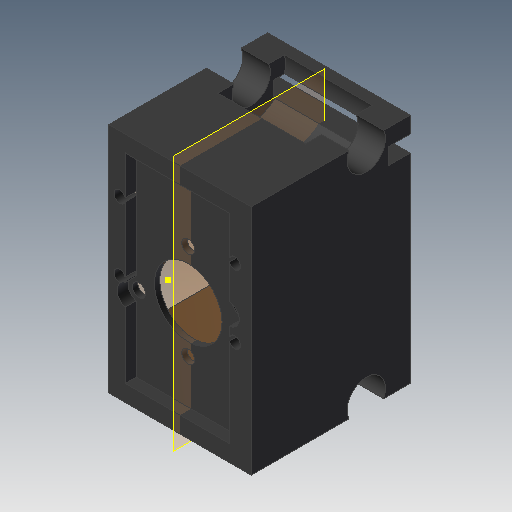
# Autodesk Inventor part: 01_Adapter_Raspicam_CCTV_lens
Saved by Autodesk Inventor 2019.4 (Build 234330000, 330)
## iProperties
Created: 2020-10-20
Part Number: 01_Adapter_Raspicam_CCTV_lens
Material: Generic
Document SubType Name: Modeling
Designer: diederichbenedict
Density: 1 g/cm^3
Appearance: Default
Author: diederichbenedict
Autodesk Inventor part; units mm, degrees
ref_plane "YZ Plane" through (0, 0, 0) normal (1, 0, 0) x (0, 1, 0)
ref_plane "XZ Plane" through (0, 0, 0) normal (0, 1, 0) x (-1, 0, 0)
ref_plane "Work Plane1" through (3.9765, -1.598, 6) normal (0, 0, 1) x (1, 0, 0)
sketch "Sketch1" plane through (3.9765, -1.598, 6) normal (0, 0, 1) x (1, 0, 0)
  arc A0 (8.7735, 0.8133) -> (8.7735, -0.0173) centre (8.2735, 0.398) ccw construction
  line L0 (8.7735, 0.8133) -> (8.7735, 2.1739) construction
  arc A1 (8.7735, 2.1739) -> (8.7735, 5.6221) centre (9.0735, 3.898) ccw construction
  line L1 (8.7735, 5.6221) -> (8.7735, 7.898) construction
  line L2 (8.7735, 7.898) -> (1.2743, 7.898) construction
  arc A2 (1.2743, 7.898) -> (-1.7274, 7.898) centre (-0.2265, 8.798) ccw construction
  line L3 (-1.7274, 7.898) -> (-8.2265, 7.898) construction
  line L4 (-8.2265, 7.898) -> (-8.2265, -1.1658) construction
  arc A3 (-8.2265, -1.1658) -> (-8.2265, -4.0381) centre (-9.2265, -2.602) ccw construction
  line L5 (-8.2265, -4.0381) -> (-8.2265, -8.102) construction
  line L6 (-8.2265, -8.102) -> (-1.9036, -8.102) construction
  arc A4 (-1.9036, -8.102) -> (1.4505, -8.102) centre (-0.2265, -8.602) ccw construction
  line L7 (1.4505, -8.102) -> (8.7735, -8.102) construction
  line L8 (8.7735, -8.102) -> (8.7735, -0.0173) construction
  line L9 (-6.2265, -6.102) -> (-6.2265, 5.898) construction
  line L10 (-6.2265, 5.898) -> (6.7735, 5.898) construction
  line L11 (6.7735, 5.898) -> (6.7735, -6.102) construction
  line L12 (6.7735, -6.102) -> (-6.2265, -6.102) construction
  circle A5 centre (-9.2265, -2.602) radius 0.9 construction
  circle A6 centre (9.0735, 3.898) radius 0.9 construction
  circle A7 centre (-0.2265, 8.798) radius 0.9 construction
  circle A8 centre (-0.2265, -8.602) radius 0.9 construction
  line L13 (10.1735, -9.602) -> (10.1735, -4.102) construction
  line L14 (12.2735, -9.602) -> (10.1735, -9.602) construction
  line L15 (12.2735, 14.398) -> (12.2735, -9.602) construction
  line L16 (-12.7265, 14.398) -> (12.2735, 14.398) construction
  line L17 (-12.7265, -9.602) -> (-12.7265, 14.398) construction
  line L18 (-10.6265, -9.602) -> (-12.7265, -9.602) construction
  line L19 (-10.6265, -4.102) -> (-10.6265, -9.602) construction
  line L20 (10.1735, -4.102) -> (-10.6265, -4.102) construction
  circle A9 centre (10.2735, 12.398) radius 1.05 construction
  circle A10 centre (10.2735, -0.102) radius 1.05 construction
  circle A11 centre (-10.7265, -0.102) radius 1.05 construction
  circle A12 centre (-10.7265, 12.398) radius 1.05 construction
  line L21 (8.7735, 0.798) -> (8.7735, 12.398) construction
  line L22 (-8.9265, 0.798) -> (8.7735, 0.798) construction
  line L23 (-8.9265, 12.398) -> (-8.9265, 0.798) construction
  line L24 (8.7735, 12.398) -> (-8.9265, 12.398) construction
  line L25 (12.2735, 14.398) -> (-12.7265, 14.398)
  line L26 (-12.7265, 14.398) -> (-12.7265, -9.602)
  line L27 (12.2735, -9.602) -> (12.2735, 14.398)
  circle A13 centre (-0.2265, 8.798) radius 1.2
  circle A14 centre (-9.2265, -2.602) radius 1.2
  circle A15 centre (-0.2265, -8.602) radius 1.2
  circle A16 centre (9.0735, 3.898) radius 1.2
  circle A17 centre (-0.2265, -0.102) radius 2.8 projected
  circle A18 centre (-0.2265, -0.102) radius 6.1789
  line L28 (-12.7265, -9.602) -> (-12.7265, -19.602)
  line L29 (-12.7265, -19.602) -> (12.2735, -19.602)
  line L30 (12.2735, -19.602) -> (12.2735, -9.602)
  line L31 (12.2735, -9.602) -> (0.4368, -9.602)
  line L32 (-0.8899, -9.602) -> (-12.7265, -9.602)
  line L33 (-12.7265, -9.602) -> (-0.8899, -9.602)
  line L34 (0.4368, -9.602) -> (12.2735, -9.602)
  line L35 (-12.7265, 14.398) -> (12.2735, 14.398)
  line L36 (12.2735, 14.398) -> (12.2735, 22.798)
  line L37 (12.2735, 22.798) -> (-12.7265, 22.798)
  line L38 (-12.7265, 22.798) -> (-12.7265, 14.398)
  line L39 (11.2735, 14.798) -> (-9.6265, 14.798) construction
  line L40 (-19.2265, -11.602) -> (11.2735, -11.602) construction
  point P0 (-3.9765, 1.598)
  dimension "d0" = 2.4
  dimension "d1" = 2.4
  dimension "d2" = 2.4
  dimension "d3" = 2.4
  dimension "d16" = 8
  dimension "d17" = 8
  constraints: 28 end point, 8 parallel, 5 centre point, 4 coincident, 4 horizontal, 4 perpendicular, 2 point on circle
  measures "d0" diameter of A13
  measures "d1" diameter of A14
  measures "d2" diameter of A15
  measures "d3" diameter of A16
  measures "d16" distance between parallel lines of L40 L29
  measures "d17" distance between parallel lines of L39 L37
extrude "Extrusion1" add sketch "Sketch1" along normal blind 1 contours L27 L31 A15 L32 L26 L25 | L25 L38 L37 L36 | L30 L29 L28 L32 A15 L31
sketch "Sketch2" plane through (3.9765, -1.598, 7) normal (0, 0, 1) x (1, 0, 0)
  circle A0 centre (-0.2265, -0.102) radius 6.1789 construction
  circle A1 centre (9.0735, 3.898) radius 1.2 construction
  circle A2 centre (-9.2265, -2.602) radius 1.2 construction
  circle A3 centre (-0.2265, 8.798) radius 1.2 construction
  line L0 (-12.7265, 22.798) -> (-12.7265, -19.602) construction
  line L1 (12.2735, -19.602) -> (12.2735, 22.798) construction
  line L2 (10.1735, -9.602) -> (10.1735, -4.102) construction
  line L3 (12.2735, -9.602) -> (10.1735, -9.602) construction
  line L4 (12.2735, 14.398) -> (12.2735, -9.602) construction
  line L5 (-12.7265, 14.398) -> (12.2735, 14.398) construction
  line L6 (-12.7265, -9.602) -> (-12.7265, 14.398) construction
  line L7 (-10.6265, -9.602) -> (-12.7265, -9.602) construction
  line L8 (-10.6265, -4.102) -> (-10.6265, -9.602) construction
  line L9 (10.1735, -4.102) -> (-10.6265, -4.102) construction
  circle A4 centre (10.2735, 12.398) radius 1.05 construction
  circle A5 centre (10.2735, -0.102) radius 1.05 construction
  circle A6 centre (-10.7265, -0.102) radius 1.05 construction
  circle A7 centre (-10.7265, 12.398) radius 1.05 construction
  line L10 (8.7735, 0.798) -> (8.7735, 12.398) construction
  line L11 (-8.9265, 0.798) -> (8.7735, 0.798) construction
  line L12 (-8.9265, 12.398) -> (-8.9265, 0.798) construction
  line L13 (8.7735, 12.398) -> (-8.9265, 12.398) construction
  line L14 (-12.7265, -19.602) -> (12.2735, -19.602) projected
  line L15 (12.2735, 22.798) -> (-12.7265, 22.798) projected
  line L16 (12.2735, 22.798) -> (-12.7265, 22.798)
  line L17 (-12.7265, 22.798) -> (-12.7265, -19.602)
  line L18 (-12.7265, -19.602) -> (12.2735, -19.602)
  line L19 (12.2735, -19.602) -> (12.2735, 22.798)
  line L20 (9.2735, 19.798) -> (-9.7265, 19.798)
  line L21 (-9.7265, 19.798) -> (-9.7265, -16.602)
  line L22 (-9.7265, -16.602) -> (9.2735, -16.602)
  line L23 (9.2735, -16.602) -> (9.2735, 19.798)
  dimension "d25" = 3
  constraints: 16 end point, 2 parallel, 1 horizontal, 1 perpendicular, 3 other
  measures "d25" distance between parallel lines of L1 L23
extrude "Extrusion2" add sketch "Sketch2" along normal blind 2
sketch "Sketch3" plane through (3.9765, -1.598, 9) normal (0, 0, 1) x (1, 0, 0)
  arc A0 (9.2735, 5.0812) -> (9.2735, 2.7148) centre (9.0735, 3.898) ccw projected
  circle A1 centre (-0.2265, 8.798) radius 1.2 projected
  arc A2 (-9.7265, -3.6929) -> (-9.7265, -1.5111) centre (-9.2265, -2.602) ccw projected
  circle A3 centre (10.2735, -0.102) radius 1.05 projected
  circle A4 centre (10.2735, 12.398) radius 1.05 projected
  circle A5 centre (-10.7265, 12.398) radius 1.05 projected
  circle A6 centre (-10.7265, -0.102) radius 1.05 projected
  circle A7 centre (-0.2265, -8.602) radius 0.9 projected
  circle A8 centre (9.0735, 3.898) radius 1.2199
  point P0 (-3.9765, 1.598)
  point P1 (8.7735, 2.7361)
  point P2 (8.7735, 5.0599)
  point P3 (-8.9265, -1.4401)
  point P4 (-10.0073, -1.6907)
  constraints: 1 centre point, 1 coincident
extrude "Extrusion3" cut sketch "Sketch3" against normal up to surface (3 mm away) contours A3 | A4 | A5 | A6 | A7 | A8
sketch "Sketch4" plane through (3.9765, -1.598, 7) normal (0, 0, 1) x (1, 0, 0)
  point P0 (-3.9765, 1.598)
sketch "Sketch5" plane through (3.9765, -1.598, 7) normal (0, 0, 1) x (1, 0, 0)
  arc A0 (9.2735, 5.1014) -> (9.2735, 2.6946) centre (9.0735, 3.898) ccw projected
  arc A1 (-9.7265, -3.6929) -> (-9.7265, -1.5111) centre (-9.2265, -2.602) ccw projected
  circle A2 centre (9.0735, 3.898) radius 2
  circle A3 centre (-9.2265, -2.602) radius 2
  point P0 (-3.9765, 1.598)
  point P1 (8.7735, 2.7156)
  point P2 (8.7735, 5.0805)
  point P3 (-8.0265, -2.602)
  point P4 (-8.0265, -2.602)
  dimension "d11" = 4
  dimension "d12" = 4
  constraints: 2 centre point, 2 coincident
  measures "d11" diameter of A2
  measures "d12" diameter of A3
extrude "Extrusion4" cut sketch "Sketch5" along normal blind 2
sketch "Sketch6" plane through (3.9765, -1.598, 6) normal (0, 0, -1) x (-1, 0, 0)
  circle A0 centre (0.2265, -0.102) radius 6.1789 projected
  circle A1 centre (9.2265, -2.602) radius 1.2 projected
  circle A2 centre (0.2265, 8.798) radius 1.2 projected
  circle A3 centre (0.2265, -8.602) radius 1.2 projected
  line L0 (12.7265, -19.602) -> (12.7265, 22.798) projected
  line L1 (12.7265, 22.798) -> (-12.2735, 22.798) projected
  line L2 (-12.2735, 22.798) -> (-12.2735, -19.602) projected
  line L3 (12.7265, -19.602) -> (-12.2735, -19.602) projected
  circle A4 centre (0.2265, -0.102) radius 8.5 construction
  line L4 (19.2265, 14.798) -> (-11.2735, 14.798) construction
  line L5 (-11.2735, 14.798) -> (-11.2735, -11.602) construction
  line L6 (-11.2735, -11.602) -> (19.2265, -11.602) construction
  line L7 (19.2265, -11.602) -> (19.2265, 14.798) construction
  line L8 (12.7265, 22.798) -> (-12.2735, 22.798) projected
  line L9 (-12.2735, 22.798) -> (-12.2735, -19.602) projected
  line L10 (12.7265, 22.798) -> (-12.2735, 22.798)
  line L11 (-12.2735, 22.798) -> (-12.2735, 14.998)
  line L12 (-12.2735, 14.998) -> (12.7265, 14.998)
  line L13 (12.7265, 14.998) -> (12.7265, 22.798)
  line L14 (12.7265, -19.602) -> (-12.2735, -19.602) projected
  line L15 (12.7265, -19.602) -> (-12.2735, -19.602)
  line L16 (-12.2735, -19.602) -> (-12.2735, -11.802)
  line L17 (-12.2735, -11.802) -> (12.7265, -11.802)
  line L18 (12.7265, -11.802) -> (12.7265, -19.602)
  point P0 (3.9765, 1.598)
  dimension "d18" = 25
  dimension "d19" = 7.8
  dimension "d20" = 7.8
  constraints: 16 end point, 4 parallel, 2 horizontal, 2 perpendicular, 2 point on line
  measures "d18" distance of L12.end L11.end
  measures "d19" distance of L11.end L10.end
  measures "d20" distance of L15.end L16.end
ref_plane "Work Plane2" through (-15.25, -13.2, -16.2) normal (0, 0, -1) x (0, 1, 0)
extrude "Extrusion5" add sketch "Sketch6" along normal blind 26 contours L3 L2 L17 L0 | L12 L2 L1 L0
sketch "Sketch7" plane through (3.9765, -1.598, 9) normal (0, 0, 1) x (1, 0, 0)
  arc A0 (9.2735, 1.908) -> (9.2735, 5.888) centre (9.0735, 3.898) ccw projected
  line L0 (9.2735, 1.908) -> (9.2735, 0.2182) projected
  arc A1 (9.2735, -0.4221) -> (9.2735, 0.2182) centre (10.2735, -0.102) ccw projected
  line L1 (9.2735, -0.4221) -> (9.2735, -16.602) projected
  line L2 (9.2735, -16.602) -> (-9.7265, -16.602) projected
  line L3 (-9.7265, -16.602) -> (-9.7265, -4.5385) projected
  arc A2 (-10.5953, -1.1438) -> (-9.7265, -4.5385) centre (-9.2265, -2.602) ccw projected
  arc A3 (-9.7265, 0.2182) -> (-10.5953, -1.1438) centre (-10.7265, -0.102) ccw projected
  line L4 (-9.7265, 0.2182) -> (-9.7265, 12.0779) projected
  arc A4 (-9.7265, 12.7182) -> (-9.7265, 12.0779) centre (-10.7265, 12.398) ccw projected
  line L5 (-9.7265, 12.7182) -> (-9.7265, 19.798) projected
  line L6 (-9.7265, 19.798) -> (9.2735, 19.798) projected
  line L7 (9.2735, 19.798) -> (9.2735, 12.7182) projected
  arc A5 (9.2735, 12.0779) -> (9.2735, 12.7182) centre (10.2735, 12.398) ccw projected
  line L8 (9.2735, 12.0779) -> (9.2735, 5.888) projected
  line L9 (-12.7265, 22.798) -> (-12.7265, -19.602) projected
  line L10 (-12.7265, -19.602) -> (12.2735, -19.602) projected
  line L11 (12.2735, -19.602) -> (12.2735, 22.798) projected
  line L12 (12.2735, 22.798) -> (-12.7265, 22.798) projected
  line L13 (12.2735, 22.798) -> (13.2735, 22.798)
  line L14 (13.2735, 22.798) -> (13.2735, -19.602)
  line L15 (13.2735, -19.602) -> (12.2735, -19.602)
  line L16 (12.2735, -19.602) -> (12.2735, 22.798)
  line L17 (-12.7265, -19.602) -> (-13.7265, -19.602)
  line L18 (-13.7265, -19.602) -> (-13.7265, 22.798)
  line L19 (-13.7265, 22.798) -> (-12.7265, 22.798)
  line L20 (-12.7265, 22.798) -> (-12.7265, -19.602)
  point P0 (-3.9765, 1.598)
  dimension "d26" = 1
  dimension "d27" = 1
  constraints: 16 end point, 4 parallel, 2 horizontal, 2 perpendicular, 1 point on line
  measures "d26" distance of L14.end L15.end
  measures "d27" distance of L18.end L19.end
extrude "Extrusion6" add sketch "Sketch7" against normal up to surface (29 mm away) contours L13 L14 L15 L11
sketch "Sketch8" plane through (17.25, -21.2, 9) normal (1, 0, 0) x (0, 0, -1)
  line L0 (0, 42.4) -> (29, 42.4) projected
  line L1 (0, 42.4) -> (0, 0) projected
  line L2 (0, 0) -> (29, 0) projected
  line L3 (3, 34.6) -> (29, 34.6) projected
  line L4 (3, 7.8) -> (29, 7.8) projected
  circle A0 centre (21, 40.9) radius 3.5
  circle A1 centre (21, 1.5) radius 3.5
  line L5 (29, 42.4) -> (29, 0) projected
  point P0 (9, 21.2)
  dimension "d30" = 7
  dimension "d31" = 7
  dimension "d34" = 1.5
  dimension "d_10" = 1.5
  constraints: 2 centre point
  measures "d30" diameter of A0
  measures "d31" diameter of A1
  measures "d34" distance from line of A1.centre L2
  measures "d_10" distance from line of L0 A0.centre
extrude "Extrusion7" cut sketch "Sketch8" against normal through all contours A0 L0 | L0 A0 | A1 L2 | L2 A1
ref_plane "Work Plane3" through (4.25, -21.2, 9) normal (1, 0, 0) x (0, 0, -1)
sketch "Sketch9" plane through (4.25, -21.2, 9) normal (1, 0, 0) x (0, 0, -1)
  circle A0 centre (21, 40.9) radius 6 projected
  line L0 (14.5, 34.4) -> (4.9, 34.4)
  arc A1 (24.1623, 0) -> (17.8377, 0) centre (21, 1.5) ccw projected
  circle A2 centre (21, 40.9) radius 6.25
  circle A3 centre (21, 1.5) radius 6.25
  point P0 (9, 21.2)
  dimension "d38" = 12.5
  dimension "d39" = 12.5
  constraints: 2 centre point, 2 coincident, 2 end point, 1 horizontal, 2 other
  measures "d38" diameter of A2
  measures "d39" diameter of A3
extrude "Extrusion8" cut sketch "Sketch9" along normal mid plane 16 contours A0 | A2 | A3
sketch "Sketch10" plane through (-8.75, -21.2, -20) normal (0, 0, -1) x (-1, 0, 0)
  line L0 (-26, 42.4) -> (0, 42.4) projected
  line L1 (-26, 0) -> (-26, 42.4) projected
  line L2 (0, 0) -> (-26, 0) projected
  line L3 (0, 7.8) -> (0, 0) projected
  line L4 (-25, 7.8) -> (0, 7.8) projected
  line L5 (-25, 34.6) -> (-25, 7.8) projected
  line L6 (0, 34.6) -> (-25, 34.6) projected
  line L7 (0, 42.4) -> (0, 34.6) projected
  line L8 (-25, 34.6) -> (0, 34.6) construction
  line L9 (-26, 37.4) -> (-26, 42.4) projected
  line L10 (0, 42.4) -> (-26, 42.4)
  line L11 (-26, 42.4) -> (-26, 39.4)
  line L12 (-26, 39.4) -> (0, 39.4)
  line L13 (0, 39.4) -> (0, 42.4)
  line L14 (-26, 34.6) -> (-26, 36.4) construction
  line L15 (-26, 36.4) -> (0, 36.4)
  line L16 (-24.7053, 7.8) -> (-25, 7.8)
  line L17 (0, 36.4) -> (-26, 36.4)
  line L18 (-26, 36.4) -> (-26, 39.4)
  line L19 (-26, 39.4) -> (0, 39.4)
  line L20 (0, 39.4) -> (0, 36.4)
  point P0 (-8.75, 21.2)
  dimension "d42" = 3
  dimension "d43" = 3
  constraints: 22 end point, 4 parallel, 4 point on line, 3 perpendicular, 2 horizontal
  measures "d42" distance of L11.end L10.end
  measures "d43" distance between parallel lines of L15 L12
extrude "Extrusion9" cut sketch "Sketch10" against normal blind 4 contours L12 L7 L15 L1
equation "\"d34\" = d_10"
body "Solid1"
